waschbaekenunterschrank (Autodesk Fusion 360 design; units mm, degrees)
Autodesk Fusion 360 part; units mm, degrees
sketch "Sketch1" plane through (0, 0, 0) normal (0, 1, 0) x (1, 0, 0)
  line L0 (0, 0) -> (0, -155)
  line L1 (-77.5, 0) -> (77.5, 0)
  line L2 (77.5, 0) -> (77.5, -155)
  line L3 (77.5, -155) -> (-77.5, -155)
  line L4 (-77.5, -155) -> (-77.5, 0)
  arc A0 (77.5, 0) -> (-77.5, 0) centre (0, 0) ccw
  line L5 (-20, -155) -> (-20, 0)
  arc A1 (20, 0) -> (-20, 0) centre (0, 0) ccw
  line L6 (20, 0) -> (20, -155)
  line L7 (-87.5, -155) -> (-87.5, 0)
  arc A2 (87.5, 0) -> (-87.5, 0) centre (0, 0) ccw
  line L8 (87.5, 0) -> (87.5, -155)
  line L9 (87.5, -155) -> (-87.5, -155)
  line L10 (-72.5, -155) -> (-72.5, 0)
  arc A3 (72.5, 0) -> (-72.5, 0) centre (0, 0) ccw
  line L11 (72.5, 0) -> (72.5, -155)
  line L12 (20, -20) -> (-20, -20)
  arc A4 (20, -20) -> (-20, -20) centre (0, -20) ccw
  dimension "d2" = 155
  dimension "d3" = 155
  dimension "d4" = 57.5
  dimension "d5" = -10
  dimension "d6" = 5
  constraint coincident L0.start A0.centre
  constraint vertical L0
  constraint perpendicular L0 L1
  constraint midpoint L0.start L1
  constraint perpendicular L1 L2
  constraint perpendicular L2 L3
  constraint perpendicular L1 L4
  constraint midpoint L0.end L3
  constraint perpendicular L7 L9
  constraint coincident L6 L12.start
  constraint coincident L5 L12.end
  constraint perpendicular L5 L12
  constraint coincident L12 A4.centre
  constraint coincident L0.start A4
  measures "d2" distance of L1.end L2.end
  measures "d3" distance of L2.end L3.end
extrude "Extrude1" add sketch "Sketch1" along normal blind 7 contours L1 L3 L4 L9 L10 | L1 A0 A3 | L1 L2 L3 L9 L11
extrude "Extrude2" add sketch "Sketch1" along normal blind 3 contours L1 L5 A4 | L1 A1 | L1 L6 A4 | L1 L3 L5 L9 L10 | L1 A1 A3 | L1 L3 L6 L9 L11 | L2 L4 A0 L7 A2 L8 L9
chamfer "Chamfer1" distance 3 angle 45 3 edges at (87.5, 0, 77.5) (0, 0, -87.5) (-87.5, 0, 77.5)
equation "d2 = 245 mm - 90 mm"
equation "d4 = ( ( 155 - 40 ) / 2 ) * 1 mm"
